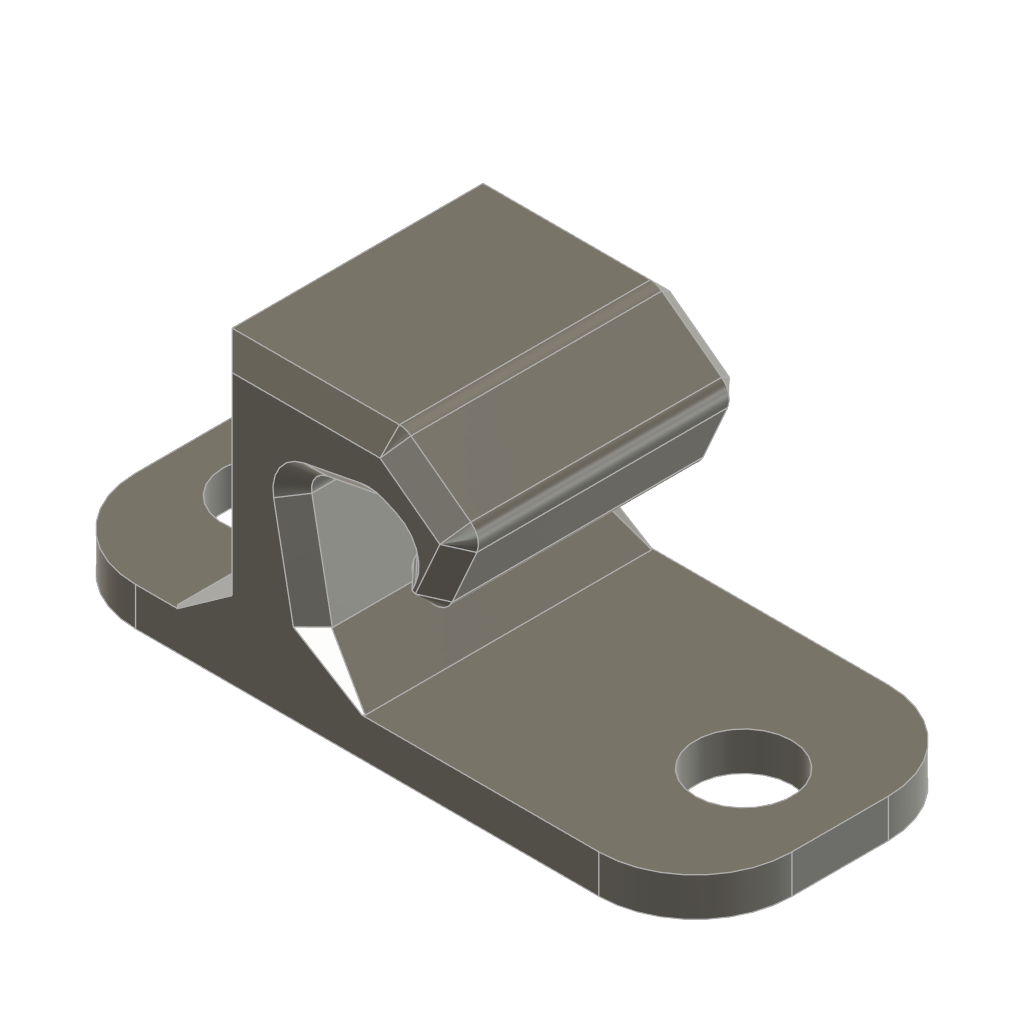
Band hook (Autodesk Fusion 360 design; units mm, degrees)
Autodesk Fusion 360 part; units mm, degrees
note: some values were not read from the file. Chosen so that the rebuilt part matches the saved one: which pieces of a blend or face edit are solid.
sketch "Sketch1" plane through (0, 0, 0) normal (0, 0, 1) x (1, 0, 0)
  line L0 (0, 0) -> (0, 15)
  line L1 (0, 15) -> (8.6667, 15)
  line L2 (9.2667, 14.8) -> (12.3626, 12.4781)
  line L3 (12.6764, 11.2719) -> (11.4061, 8.4138)
  line L4 (10.0862, 7.9061) -> (9.9138, 7.9828)
  line L5 (9.4061, 9.3027) -> (9.5939, 9.7251)
  line L6 (9.0862, 11.045) -> (8.4507, 11.3275)
  line L7 (7.8546, 11.3955) -> (4.9237, 10.8285)
  line L8 (4.1318, 9.6567) -> (6, 0)
  line L9 (6, 0) -> (0, 0)
  arc A0 (4.9237, 10.8285) -> (4.1318, 9.6567) centre (5.1136, 9.8467) ccw
  arc A1 (8.4507, 11.3275) -> (7.8546, 11.3955) centre (8.0446, 10.4137) ccw
  arc A2 (9.5939, 9.7251) -> (9.0862, 11.045) centre (8.6801, 10.1312) ccw
  arc A3 (9.4061, 9.3027) -> (9.9138, 7.9828) centre (10.32, 8.8966) ccw
  arc A4 (10.0862, 7.9061) -> (11.4061, 8.4138) centre (10.4923, 8.82) ccw
  arc A5 (12.6764, 11.2719) -> (12.3626, 12.4781) centre (11.7626, 11.6781) ccw
  arc A6 (9.2667, 14.8) -> (8.6667, 15) centre (8.6667, 14) ccw
  line L10 (-9, 0) -> (25, 0)
  line L11 (25, 0) -> (25, 2)
  line L12 (25, 2) -> (-9, 2)
  line L13 (-9, 2) -> (-9, 0)
  dimension "d1" = 15
  dimension "d2" = 1
  constraint coincident L0.start L9.end
  constraint vertical L0
  constraint perpendicular L0 L1
  constraint perpendicular L3 L4
  constraint perpendicular L4 L5
  constraint perpendicular L5 L6
  constraint perpendicular L7 L8
  constraint tangent L7 A0
  constraint tangent L8 A0
  constraint tangent L6 A1
  constraint tangent L7 A1
  constraint equal A0 A1
  constraint tangent L5 A2
  constraint tangent L6 A2
  constraint equal A0 A2
  constraint tangent L4 A3
  constraint tangent L5 A3
  constraint equal A0 A3
  constraint tangent L3 A4
  constraint tangent L4 A4
  constraint equal A0 A4
  constraint tangent L2 A5
  constraint tangent L3 A5
  constraint equal A0 A5
  constraint tangent L1 A6
  constraint tangent L2 A6
  constraint equal A0 A6
  constraint horizontal L10
  constraint vertical L11
  constraint horizontal L12
  constraint vertical L13
  measures "d1" distance of L0.start L0.end
  measures "d2" radius of A0
extrude "Extrude1" add sketch "Sketch1" along normal blind 15
chamfer "Chamfer1" distance 1 angle 45 32 edges at (0, 8.5, 15) (4.3333, 15, 15) (4.8725, 5.8284, 15) (4.2851, 10.4066, 15) (6.3892, 11.112, 15) (8.1579, 11.4072, 15) (8.7684, 11.1862, 15) (9.6134, 10.4902, 15) (9.5, 9.5139, 15) (9.3866, 8.5376, 15) (10, 7.9444, 15) (10.8513, 7.8866, 15) (12.0413, 9.8429, 15) (12.7304, 11.9298, 15) (10.8146, 13.639, 15) (8.9829, 14.9487, 15) (4.3333, 15, 0) (8.9829, 14.9487, 0) (10.8146, 13.639, 0) (12.7304, 11.9298, 0) (12.0413, 9.8429, 0) (10.8513, 7.8866, 0) (10, 7.9444, 0) (9.3866, 8.5376, 0) (9.5, 9.5139, 0) (9.6134, 10.4902, 0) (8.7684, 11.1862, 0) (8.1579, 11.4072, 0) (6.3892, 11.112, 0) (4.2851, 10.4066, 0) (4.8725, 5.8284, 0) (0, 8.5, 0)
hole "Hole1" at (20, 2, 7.5) direction (0, -1, 0) diameter 5 depth 10 tip angle 118
hole "Hole2" at (-4.4645, 2, 7.5) direction (0, -1, 0) diameter 5 depth 10 tip angle 118
fillet "Fillet1" radius 5 4 edges at (-9, 1, 15) (-9, 1, 0) (25, 1, 15) (25, 1, 0)
chamfer "Chamfer2" distance 2.2 angle 45 3 edges at (5.6131, 2, 7.5) (5.1038, 2, 0.5) (5.1038, 2, 14.5)
chamfer "Chamfer2" distance 2 angle 45 3 edges at (0, 2, 7.5) (0.5, 2, 14.5) (0.5, 2, 0.5)
